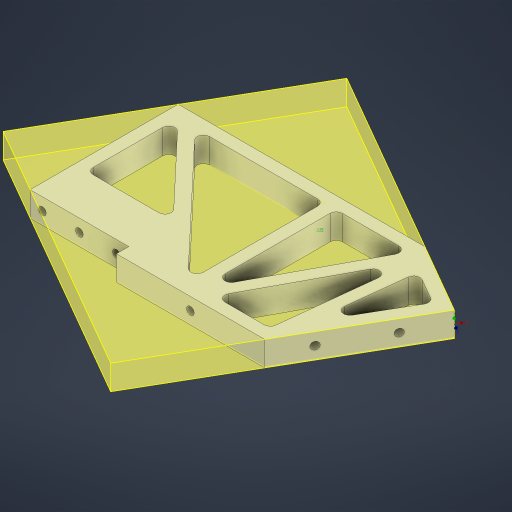
# Autodesk Inventor part: Third Baseplate
Saved by Autodesk Inventor 2023 (Build 270158000, 158)
## iProperties
Created: 2022-05-02
Part Number: Third Baseplate
Material: Generic
Document SubType Name: Modeling
Designer: FizzyApple12
Density: 1 g/cm^3
Appearance: Default
Author: FizzyApple12
Autodesk Inventor part; units mm, degrees
ref_plane "YZ Plane" through (0, 0, 0) normal (1, 0, 0) x (0, 1, 0)
ref_plane "XZ Plane" through (0, 0, 0) normal (0, 1, 0) x (-1, 0, 0)
ref_plane "XY Plane" through (0, 0, 0) normal (0, 0, 1) x (1, 0, 0)
sketch "Sketch1" plane through (0, 0, 0) normal (0, 0, 1) x (1, 0, 0)
  line L0 (0, 0) -> (50.8, 0)
  line L1 (50.8, 0) -> (50.8, 12.7)
  line L2 (50.8, 12.7) -> (0, 12.7)
  line L3 (0, 12.7) -> (0, 0)
  dimension "d0" = 50.8
  dimension "d1" = 12.7
  constraints: 8 end point, 2 parallel, 1 horizontal, 1 perpendicular
  measures "d0" distance of L2.end L1.end
  measures "d1" distance of L1.end L0.end
extrude "Extrusion1" add sketch "Sketch1" along normal blind 76.2
sketch "Sketch2" plane through (0, 0, 76.2) normal (0, 0, 1) x (1, 0, 0)
  line L0 (50.8, 12.7) -> (0, 12.7) construction
  line L1 (50.8, 0) -> (50.8, 12.7) construction
  line L2 (0, 12.7) -> (50.8, 12.7) construction
  line L3 (50.8, 12.7) -> (50.8, 6.35) construction
  line L4 (50.8, 6.35) -> (0, 6.35) construction
  line L5 (0, 6.35) -> (0, 12.7) construction
  point P0 (0, 0)
  point P1 (25.4, 6.35)
  point P2 (6.35, 6.35)
  point P3 (44.45, 6.35)
  dimension "d4" = 6.35
  dimension "d5" = 19.05
  dimension "d6" = 19.05
  constraints: 8 end point, 2 midpoint, 2 parallel, 2 point on line, 1 horizontal, 1 perpendicular
  measures "d4" distance of L2.end L3.end
  measures "d5" distance of point (6.35, 6.35) point (25.4, 6.35)
  measures "d6" distance of point (44.45, 6.35) point (25.4, 6.35)
hole "Hole1" at (25.4, 6.35, 76.2) at (6.35, 6.35, 76.2) at (44.45, 6.35, 76.2) direction (0, 0, -1) diameter 3.9624 depth 16.51 thread size "10-32 UNF" class "2B" standard "ANSI Unified Screw Threads"
sketch "Sketch3" plane through (50.8, 0, 0) normal (1, 0, 0) x (0, 0, -1)
  line L0 (0, 0) -> (-76.2, 0) projected
  line L1 (-76.2, 0) -> (-76.2, 12.7) projected
  line L2 (0, 0) -> (-76.2, 0)
  line L3 (-76.2, 0) -> (-76.2, 12.7)
  line L4 (-76.2, 12.7) -> (0, 12.7)
  line L5 (0, 12.7) -> (0, 0)
  constraints: 8 end point, 2 parallel, 1 horizontal, 1 perpendicular
extrude "Extrusion2" add sketch "Sketch3" along normal blind 76.2
sketch "Sketch4" plane through (0, 0, 76.2) normal (0, 0, 1) x (1, 0, 0)
  line L0 (0, 12.7) -> (127, 12.7) projected
  line L1 (0, 0) -> (127, 0) projected
  line L2 (127, 12.7) -> (50.8, 12.7)
  line L3 (50.8, 12.7) -> (50.8, 0)
  line L4 (50.8, 0) -> (127, 0)
  line L5 (127, 0) -> (127, 12.7)
  dimension "d16" = 76.2
  constraints: 8 end point, 2 parallel, 1 horizontal, 1 perpendicular, 1 point on line
  measures "d16" distance of L4.end L3.end
extrude "Extrusion3" add sketch "Sketch4" along normal blind 6.35
sketch "Sketch5" plane through (0, 0, 0) normal (0, -1, 0) x (1, 0, 0)
  line L0 (127, 0) -> (162.7452, 20.6375)
  line L1 (127, 0) -> (168.275, 0) construction
  line L2 (127, 0) -> (127, 82.55) projected
  line L3 (162.7452, 20.6375) -> (127, 82.55)
  line L4 (127, 82.55) -> (127, 0)
  point P0 (0, 0)
  dimension "d19" = 41.275
  dimension "d20" = 30
  constraints: 8 end point, 1 collinear, 1 equal length, 1 horizontal
  measures "d19" distance of L0.start L0.end
  measures "d20" angle of L1 L0
extrude "Extrusion4" add sketch "Sketch5" against normal up to surface (12.7 mm away)
sketch "Sketch6" plane through (0, 0, 76.2) normal (0, 1, 0) x (1, 0, 0)
  line L0 (4.3688, 16.51) -> (8.3312, 16.51) projected
  line L1 (8.3312, 0) -> (4.3688, 0) projected
  line L2 (8.3312, 0) -> (4.3688, 0) projected
  line L3 (4.3688, 16.51) -> (8.3312, 16.51) projected
  line L4 (0, 76.2) -> (0, 0) projected
  line L5 (0, 16.51) -> (50.8, 16.51)
  line L6 (50.8, 0) -> (50.8, -6.35) projected
  line L7 (50.8, 16.51) -> (50.8, 0)
  line L8 (0, 76.2) -> (127, 76.2) projected
  line L9 (6.35, 22.86) -> (6.35, 69.85)
  line L10 (6.35, 69.85) -> (50.8, 22.86)
  line L11 (50.8, 22.86) -> (6.35, 22.86)
  line L12 (57.15, 16.1471) -> (57.15, 0)
  line L13 (57.15, 0) -> (72.4243, 0)
  line L14 (72.4243, 0) -> (57.15, 16.1471)
  line L15 (127, -6.35) -> (50.8, -6.35) projected
  line L16 (6.35, 69.85) -> (10.9631, 74.2137) construction
  line L17 (10.9631, 74.2137) -> (15.0909, 69.85) construction
  line L18 (15.0909, 69.85) -> (81.4011, -0.2494)
  line L19 (81.4011, -0.2494) -> (81.4011, 69.85)
  line L20 (81.4011, 69.85) -> (15.0909, 69.85)
  line L21 (127, 76.2) -> (162.7452, 55.5625) projected
  line L22 (72.4243, 0) -> (77.0374, 4.3637) construction
  line L23 (77.0374, 4.3637) -> (81.4011, -0.2494) construction
  line L24 (87.7511, 0) -> (87.7511, 69.85)
  line L25 (87.7511, 69.85) -> (125.2985, 69.85)
  line L26 (125.2985, 69.85) -> (87.7511, 0)
  line L27 (130.8003, 66.6735) -> (94.9604, 0)
  line L28 (94.9604, 0) -> (123.3338, 0)
  line L29 (123.3338, 0) -> (130.8003, 66.6735)
  line L30 (162.7452, 55.5625) -> (127, -6.35) projected
  line L31 (136.802, 63.2085) -> (154.0709, 53.2382)
  line L32 (154.0709, 53.2382) -> (131.2611, 13.7305)
  line L33 (131.2611, 13.7305) -> (136.802, 63.2085)
  point P0 (6.35, 16.51)
  point P1 (57.15, 8.0736)
  point P2 (145.4365, 58.2234)
  dimension "d23" = 50.8
  dimension "d24" = 6.35
  dimension "d25" = 6.35
  dimension "d26" = 6.35
  dimension "d27" = 6.35
  dimension "d28" = 0
  dimension "d29" = 6.35
  dimension "d30" = 6.35
  dimension "d31" = 6.35
  dimension "d33" = 6.35
  dimension "d34" = 6.35
  dimension "d39" = 6.35
  dimension "d40" = 6.35
  dimension "d41" = 6.35
  dimension "d42" = 6.35
  dimension "d43" = 6.35
  dimension "d44" = 6.35
  dimension "d45" = 6.35
  dimension "d46" = 6.35
  dimension "d47" = 6.35
  dimension "d48" = 6.35
  dimension "d49" = 6.35
  dimension "d50" = 6.35
  dimension "d51" = 6.35
  constraints: 48 end point, 7 parallel, 6 perpendicular, 4 point on line, 3 midpoint, 2 vertical, 1 collinear, 1 horizontal
  measures "d23" distance of L5.start L5.end
  measures "d24" distance from line of L5 L9.start
  measures "d25" distance from line of L4 L9.start
  measures "d26" distance from line of L8 L9.end
  measures "d27" distance from line of L9.end L4
  measures "d28" distance from line of L7 L10.end
  measures "d29" distance from line of L5 L10.end
  measures "d30" distance from line of point (57.15, 8.074) L7
  measures "d31" distance between parallel lines of L15 L13
  measures "d33" distance of L9.end L16.end
  measures "d34" distance between parallel lines of L8 L20
  measures "d39" distance of L13.end L22.end
  measures "d40" distance of L22.end L18.end
  measures "d41" distance between parallel lines of L19 L24
  measures "d42" distance from line of L8 L24.end
  measures "d43" distance from line of L15 L24.start
  measures "d44" distance from line of L21 L25.end
  measures "d45" distance between parallel lines of L15 L28
  measures "d46" distance between parallel lines of L26 L27
  measures "d47" distance from line of L21 L27.start
  measures "d48" distance from line of L30 L28.end
  measures "d49" distance between parallel lines of L29 L33
  measures "d50" distance from line of L21 point (145.436, 58.223)
  measures "d51" distance between parallel lines of L30 L32
extrude "Extrusion5" cut sketch "Sketch6" along normal through all contours L9 L10 L11 | L20 L19 L18 | L24 L25 L26 | L29 L28 L27 | L31 L32 L33
fillet "Fillet1" radius 3.175 15 edges at (130.8003, 6.35, 9.5265) (136.802, 6.35, 12.9915) (154.0709, 6.35, 22.9618) (131.2611, 6.35, 62.4695) (94.9604, 6.35, 76.2) (123.3338, 6.35, 76.2) (125.2985, 6.35, 6.35) (87.7511, 6.35, 6.35) (87.7511, 6.35, 76.2) (81.4011, 6.35, 76.4494) (81.4011, 6.35, 6.35) (15.0909, 6.35, 6.35) (6.35, 6.35, 53.34) (50.8, 6.35, 53.34) (6.35, 6.35, 6.35)
sketch "Sketch7" plane through (0, 0, 82.55) normal (0, 0, 1) x (1, 0, 0)
  line L0 (127, 0) -> (127, 12.7) construction
  line L1 (127, 6.35) -> (50.8, 6.35) construction
  line L2 (50.8, 12.7) -> (50.8, 0) construction
  point P0 (0, 0)
  point P1 (88.9, 6.35)
  constraints: 3 midpoint, 2 end point
hole "Hole2" at (88.9, 6.35, 82.55) direction (0, 0, -1) diameter 3.9624 depth 8.89 thread size "10-32 UNF" class "2B" standard "ANSI Unified Screw Threads"
sketch "Sketch8" plane through (127, 0, 82.55) normal (0.8660254, 0, 0.5) x (0.5, 0, -0.8660254)
  line L0 (0, 0) -> (0, 12.7) construction
  line L1 (71.4904, 0) -> (71.4904, 12.7) construction
  line L2 (61.9654, 12.7) -> (34.7119, 12.7) construction
  point P0 (7.9904, 0)
  point P1 (19.05, 6.35)
  point P2 (50.8, 6.35)
  dimension "d69" = 19.05
  dimension "d70" = 31.75
  measures "d69" distance from line of point (19.05, 6.35) L0
  measures "d70" distance of point (50.8, 6.35) point (19.05, 6.35)
hole "Hole3" at (136.525, 6.35, 66.0522) at (152.4, 6.35, 38.5559) direction (-0.8660254, 0, -0.5) diameter 3.9624 depth 8.89 thread size "10-32 UNF" class "2B" standard "ANSI Unified Screw Threads"
sketch "Sketch9" plane through (0, 0, 0) normal (-1, 0, 0) x (0, 0, 1)
  line L0 (0, 12.7) -> (0, 0) construction
  line L1 (0, 6.35) -> (76.2, 6.35) construction
  point P0 (19.05, 6.35)
  point P1 (44.45, 6.35)
  point P2 (31.75, 6.35)
  dimension "d71" = 25.4
  dimension "d72" = 19.05
  dimension "d73" = 12.7
  constraints: 3 point on line, 2 end point, 1 horizontal, 1 midpoint
  measures "d71" distance of point (44.45, 6.35) point (19.05, 6.35)
  measures "d72" distance from line of L0 point (19.05, 6.35)
  measures "d73" distance of point (31.75, 6.35) point (19.05, 6.35)
hole "Hole4" [suppressed]
chamfer "Chamfer1" [suppressed]
sketch "Sketch10" plane through (0, 0, 0) normal (0, -1, 0) x (1, 0, 0)
  line L0 (78.2261, 6.35) -> (22.4648, 6.35) construction
  line L1 (78.2261, 6.35) -> (81.4011, 6.35) construction
  arc A0 (78.2261, 6.35) -> (81.4011, 9.525) centre (78.2261, 9.525) ccw construction
  line L2 (81.4011, 6.35) -> (81.4011, 9.525) construction
  point P0 (0, 0)
  dimension "d84" = 3.175
  constraints: 4 end point, 1 coincident, 1 collinear
  measures "d84" distance of L0.start L1.end
sketch "Sketch11" plane through (0, 12.7, 76.2) normal (0, 1, 0) x (1, 0, 0)
  line L0 (78.2261, 69.85) -> (81.4011, 69.85) construction
  line L1 (81.4011, 69.85) -> (81.4011, 66.675) construction
  point P0 (0, 76.2)
body "Solid1"
